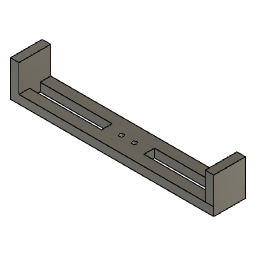
limitMechanism v1 (Autodesk Fusion 360 design; units mm, degrees)
Autodesk Fusion 360 part; units mm, degrees
sketch "Sketch1" plane through (0, 0, 0) normal (0, 0, 1) x (1, 0, 0)
  line L0 (10, -7.5) -> (-10, -7.5)
  line L1 (-10, -7.5) -> (-10, 7.5)
  line L2 (-10, 7.5) -> (10, 7.5)
  line L3 (10, 7.5) -> (10, -7.5)
  line L4 (10, -7.5) -> (-10, 7.5) construction
  line L5 (-10, -7.5) -> (10, 7.5) construction
  line L6 (0, 0) -> (0, 7) construction
  dimension "d1" = 20
  dimension "d2" = 15
  constraint horizontal L0
  constraint perpendicular L0 L1
  constraint parallel L0 L2
  constraint parallel L1 L3
  constraint coincident L4 L6.start
  constraint coincident L5 L6.start
  constraint coincident L6.start origin
  constraint vertical L6
  measures "d1" distance of L1.end L2.end
  measures "d2" distance of L0.end L1.end
extrude "Extrude1" add sketch "Sketch1" along normal blind 4
sketch "Sketch2" plane through (0, 0, 4) normal (0, 0, 1) x (-1, 0, 0)
  line L0 (-10, -7.5) -> (10, -7.5)
  line L1 (10, -7.5) -> (10, 7.5)
  line L2 (10, 7.5) -> (-10, 7.5)
  line L3 (-10, 7.5) -> (-10, -7.5)
  line L4 (10, 7.5) -> (-10, -7.5) construction
  line L5 (-10, 7.5) -> (10, -7.5) construction
  line L6 (0, 0) -> (-3, 0) construction
  circle A0 centre (-3, 0) radius 1
  line L7 (0, 0) -> (3, 0) construction
  circle A1 centre (3, 0) radius 1
  dimension "d5" = 3
  dimension "d6" = 2
  dimension "d7" = 3
  dimension "d8" = 2
  constraint coincident L1.end L2.start
  constraint coincident L0.start L3.end
  constraint coincident L2.end L3.start
  constraint coincident L0.end L1.start
  constraint coincident L6.start L7.start
  constraint horizontal L6
  constraint coincident L6.end A0.centre
  constraint parallel L6 L7
  constraint coincident L7.end A1.centre
  measures "d5" distance of L6.start L6.end
  measures "d6" diameter of A0
  measures "d7" distance of L6.start L7.end
  measures "d8" diameter of A1
extrude "Extrude2" cut sketch "Sketch2" against normal up to surface (4 mm away) contours A0 | A1
ref_plane "WorkPlane1" through (48, 0, 2) normal (1, 0, 0) x (0, 1, 0)
sketch "Sketch3" plane through (48, 0, 2) normal (1, 0, 0) x (0, 1, 0)
  line L0 (-7.5, 2) -> (-2.5, 2)
  line L1 (-2.5, 2) -> (-2.5, -2)
  line L2 (-2.5, -2) -> (-7.5, -2)
  line L3 (-7.5, -2) -> (-7.5, 2)
  line L4 (7.5, 2) -> (2.5, 2)
  line L5 (2.5, 2) -> (2.5, -2)
  line L6 (2.5, -2) -> (7.5, -2)
  line L7 (7.5, -2) -> (7.5, 2)
  constraint horizontal L0
  constraint vertical L1
  constraint horizontal L2
  constraint vertical L3
  constraint horizontal L4
  constraint vertical L5
  constraint horizontal L6
  constraint vertical L7
extrude "Extrude3" add sketch "Sketch3" against normal up to surface (38 mm away)
sketch "Sketch4" plane through (0, -2.5, 0) normal (0, 1, 0) x (-1, 0, 0)
  line L0 (-10, 0) -> (-10, 4)
  line L1 (-10, 4) -> (-48, 4)
  line L2 (-48, 4) -> (-48, 0)
  line L3 (-48, 0) -> (-10, 0)
  line L4 (-48, 4) -> (-44, 4)
  line L5 (-44, 4) -> (-44, 0)
  line L6 (-44, 0) -> (-48, 0)
  line L7 (-48, 0) -> (-48, 4)
  constraint coincident L1.end L2.start
  constraint coincident L1 L4.end
  constraint perpendicular L2 L4
  constraint coincident L3 L5.end
  constraint perpendicular L3 L5
  constraint coincident L2.end L3.start
  constraint perpendicular L2 L6
extrude "Extrude4" add sketch "Sketch4" along normal up to surface (5 mm away) contours L1 L2 L3 L4 L5 L6 L7
sketch "Sketch5" plane through (0, 0, 4) normal (0, 0, 1) x (-1, 0, 0)
  line L0 (-44, 2.5) -> (-10, 2.5)
  line L1 (-10, 2.5) -> (-10, -2.5)
  line L2 (-10, -2.5) -> (-44, -2.5)
  line L3 (-44, -2.5) -> (-44, 2.5)
  circle A0 centre (3, 0) radius 1
  circle A1 centre (-3, 0) radius 1
  line L4 (-48, 7.5) -> (-48, -7.5)
  line L5 (-48, -7.5) -> (10, -7.5)
  line L6 (10, -7.5) -> (10, 7.5)
  line L7 (10, 7.5) -> (-48, 7.5)
  line L8 (-44, -2.5) -> (-44, -7.5)
  line L9 (-44, 2.5) -> (-44, 7.5)
  constraint coincident L2.end L3.start
  constraint coincident L5 L8.end
  constraint perpendicular L5 L8
  constraint coincident L0.start L3.end
  constraint coincident L7 L9.end
  constraint perpendicular L7 L9
extrude "Extrude5" add sketch "Sketch5" along normal blind 13 contours L3 L4 L5 L7 L8 L9
ref_plane "WorkPlane2" through (-48, 0, 2) normal (-1, 0, 0) x (0, -1, 0)
sketch "Sketch6" plane through (-48, 0, 2) normal (-1, 0, 0) x (0, 1, 0)
  line L0 (7.5, -2) -> (2.5, -2)
  line L1 (2.5, -2) -> (2.5, 2)
  line L2 (2.5, 2) -> (7.5, 2)
  line L3 (7.5, 2) -> (7.5, -2)
  line L4 (-7.5, -2) -> (-2.5, -2)
  line L5 (-2.5, -2) -> (-2.5, 2)
  line L6 (-2.5, 2) -> (-7.5, 2)
  line L7 (-7.5, 2) -> (-7.5, -2)
  constraint horizontal L0
  constraint vertical L1
  constraint horizontal L2
  constraint vertical L3
  constraint horizontal L4
  constraint vertical L5
  constraint horizontal L6
  constraint vertical L7
extrude "Extrude6" add sketch "Sketch6" against normal up to surface (38 mm away)
sketch "Sketch7" plane through (0, 2.5, 0) normal (0, -1, 0) x (1, 0, 0)
  line L0 (-10, 0) -> (-10, 4)
  line L1 (-10, 4) -> (-48, 4)
  line L2 (-48, 4) -> (-48, 0)
  line L3 (-48, 0) -> (-10, 0)
  line L4 (-48, 4) -> (-44, 4)
  line L5 (-44, 4) -> (-44, 0)
  line L6 (-44, 0) -> (-48, 0)
  line L7 (-48, 0) -> (-48, 4)
  constraint coincident L1.end L2.start
  constraint coincident L1 L4.end
  constraint perpendicular L2 L4
  constraint coincident L3 L5.end
  constraint perpendicular L3 L5
  constraint coincident L2.end L3.start
  constraint perpendicular L5 L6
extrude "Extrude7" add sketch "Sketch7" along normal up to surface (5 mm away) contours L1 L2 L3 L4 L5 L6 L7
sketch "Sketch8" plane through (0, 0, 4) normal (0, 0, 1) x (-1, 0, 0)
  line L0 (44, -2.5) -> (10, -2.5)
  line L1 (10, -2.5) -> (10, 2.5)
  line L2 (10, 2.5) -> (44, 2.5)
  line L3 (44, 2.5) -> (44, -2.5)
  circle A0 centre (-3, 0) radius 1
  circle A1 centre (3, 0) radius 1
  line L4 (48, -7.5) -> (48, 7.5)
  line L5 (48, 7.5) -> (-44, 7.5)
  line L6 (-44, 7.5) -> (-44, 2.5)
  line L7 (-44, 2.5) -> (-10, 2.5)
  line L8 (-10, 2.5) -> (-10, -2.5)
  line L9 (-10, -2.5) -> (-44, -2.5)
  line L10 (-44, -2.5) -> (-44, -7.5)
  line L11 (-44, -7.5) -> (48, -7.5)
  line L12 (44, 2.5) -> (44, 7.5)
  line L13 (44, -2.5) -> (44, -7.5)
  constraint coincident L2.end L3.start
  constraint coincident L5 L12.end
  constraint perpendicular L5 L12
  constraint coincident L0.start L3.end
  constraint coincident L11 L13.end
  constraint perpendicular L11 L13
extrude "Extrude8" add sketch "Sketch8" along normal blind 13 contours L3 L4 L5 L11 L12 L13
